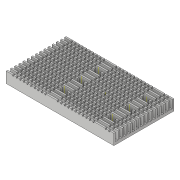
# Autodesk Inventor part: 6089-107-RevA_HEATSINK_VU7P
Saved by Autodesk Inventor 2017.3 (Build 213256000, 256)
## iProperties
Created: 2019-01-23
Part Number: 6089-107-RevA_HEATSINK_VU7P
Material: Generic
Document SubType Name: Modeling
Designer: crs5
Density: 1 g/cm^3
Appearance: Default
Author: crs5
Autodesk Inventor part; units mm, degrees
ref_plane "YZ Plane" through (0, 0, 0) normal (1, 0, 0) x (0, 1, 0)
ref_plane "XZ Plane" through (0, 0, 0) normal (0, 1, 0) x (-1, 0, 0)
ref_plane "XY Plane" through (0, 0, 0) normal (0, 0, 1) x (1, 0, 0)
sketch "Sketch1" plane through (0, 0, 0) normal (0, 1, 0) x (-1, 0, 0)
  line L0 (0, 0) -> (150, 0)
  line L1 (150, 0) -> (150, -83.5)
  line L2 (150, -83.5) -> (0, -83.5)
  line L3 (0, -83.5) -> (0, 0)
  dimension "d0" = 83.5
  dimension "d1" = 150
  constraints: 8 end point, 2 parallel, 1 horizontal, 1 perpendicular
  measures "d0" distance of L2.end L0.start
  measures "d1" distance of L0.start L0.end
extrude "Extrusion1" add sketch "Sketch1" along normal blind 15
hole "Hole1" at (-20, 15, -18.5214) direction (0, -1, 0) diameter 6 end through all counterbore diameter 8.9 counterbore depth 13.5
pattern_linear "Rectangular Pattern1" count 3 spacing 23.2286 along (0, 0, -1) count 2 spacing 67 along (-1, 0, 0) of "Hole1"
hole "Hole2" at (-53.5, 15, -41.75) direction (0, -1, 0) diameter 1.8 end through all
sketch "Sketch2" plane through (0, 0, 0) normal (1, 0, 0) x (0, 0, -1)
  line L0 (0, 15) -> (83.5, 15) projected
  line L1 (2.2, 15) -> (5.8071, 15)
  line L2 (5.8071, 15) -> (5.8071, 4)
  line L3 (5.8071, 4) -> (2.2, 4)
  line L4 (2.2, 4) -> (2.2, 15)
  line L5 (83.5, 0) -> (0, 0) projected
  line L6 (0, 0) -> (0, 15) projected
  dimension "d28" = 4
  dimension "d29" = 2.2
  dimension "d30" = 3.6071
  constraints: 8 end point, 2 parallel, 1 horizontal, 1 perpendicular, 1 point on line
  measures "d28" distance between parallel lines of L5 L3
  measures "d29" distance between parallel lines of L6 L4
  measures "d30" distance of L2.end L3.end
extrude "Extrusion2" cut sketch "Sketch2" against normal up to next
pattern_linear "Rectangular Pattern2" count 14 spacing 5.8071 along (0, 0, -1) of "Extrusion2"
sketch "Sketch3" plane through (-150, 0, 0) normal (0, 0, 1) x (1, 0, 0)
  line L0 (150, 15) -> (0, 15) projected
  line L1 (120.8, 15) -> (122.3, 15)
  line L2 (122.3, 15) -> (122.3, 13.5)
  line L3 (122.3, 13.5) -> (120.8, 13.5)
  line L4 (120.8, 13.5) -> (120.8, 15)
  line L5 (150, 0) -> (150, 15) projected
  dimension "d36" = 1.5
  dimension "d37" = 1.5
  dimension "d38" = 27.7
  constraints: 8 end point, 2 parallel, 1 horizontal, 1 perpendicular, 1 point on line
  measures "d36" distance of L1.end L2.end
  measures "d37" distance of L2.end L3.end
  measures "d38" distance between parallel lines of L2 L5
extrude "Extrusion3" cut sketch "Sketch3" against normal blind 83.5
pattern_linear "Rectangular Pattern3" count 11 spacing 5 along (-1, 0, 0) of "Extrusion3"
sketch "Sketch4" plane through (-150, 0, 0) normal (0, 0, 1) x (1, 0, 0)
  line L0 (150, 15) -> (122.3, 15) projected
  line L1 (137.7, 15) -> (139.2, 15)
  line L2 (139.2, 15) -> (139.2, 13.5)
  line L3 (139.2, 13.5) -> (137.7, 13.5)
  line L4 (137.7, 13.5) -> (137.7, 15)
  line L5 (150, 0) -> (150, 15) projected
  dimension "d44" = 1.5
  dimension "d45" = 1.5
  dimension "d46" = 12.3
  constraints: 8 end point, 2 parallel, 1 horizontal, 1 perpendicular, 1 point on line
  measures "d44" distance of L1.end L2.end
  measures "d45" distance of L2.end L3.end
  measures "d46" distance between parallel lines of L5 L4
extrude "Extrusion4" cut sketch "Sketch4" against normal blind 83.5
pattern_linear "Rectangular Pattern4" count 2 spacing 5 along (1, 0, 0) of "Extrusion4"
sketch "Sketch6" plane through (-150, 0, 0) normal (0, 0, 1) x (1, 0, 0)
  line L0 (0, 15) -> (70.8, 15) projected
  line L1 (53.8, 15) -> (55.3, 15)
  line L2 (55.3, 15) -> (55.3, 13.5)
  line L3 (55.3, 13.5) -> (53.8, 13.5)
  line L4 (53.8, 13.5) -> (53.8, 15)
  line L5 (150, 0) -> (150, 15) projected
  dimension "d52" = 1.5
  dimension "d53" = 1.5
  dimension "d54" = 94.7
  constraints: 8 end point, 2 parallel, 1 horizontal, 1 perpendicular, 1 point on line
  measures "d52" distance of L1.end L2.end
  measures "d53" distance of L2.end L3.end
  measures "d54" distance between parallel lines of L5 L2
extrude "Extrusion5" cut sketch "Sketch6" against normal blind 83.5
pattern_linear "Rectangular Pattern5" count 10 spacing 5 along (-1, 0, 0) of "Extrusion5"
equation "\"d0\" = hs_width"
equation "\"d1\" = hs_length_VU7P"
equation "\"d2\" = hs_overall_height"
equation "\"d6\" = hole_dia"
equation "\"d4\" = hole_ll_x"
equation "\"d5\" = hole_ll_y"
equation "\"d8\" = spring_hole_ID"
equation "\"d9\" = spring_hole_total_depth"
equation "\"d15\" = hole_lc_x - hole_ll_x"
equation "\"d18\" = hole_ul_y - hole_ll_y"
equation "\"d19\" = hole_fpga_center_x"
equation "\"d20\" = hole_fpga_center_y"
equation "\"d23\" = spring_hole_ID"
equation "\"d24\" = spring_hole_total_depth"
equation "\"d28\" = hs_base_thickness"
equation "\"d29\" = hs_fin_thickness"
equation "\"d30\" = hs_fin_gap"
equation "\"d31\" = hs_overall_height"
equation "\"d35\" = hs_pitch"
equation "\"d39\" = hs_width"
equation "\"d47\" = hs_width"
equation "\"d55\" = hs_width"
equation "\"hs_length_VU7P\" = 150"
equation "\"hs_length_KU15P\" = 125"
equation "\"hs_width\" = 83.5"
equation "\"hs_base_thickness\" = 4"
equation "\"hs_overall_height\" = 15"
equation "\"hs_fin_thickness\" = 2.2"
equation "\"hole_y_spacing\" = 67"
equation "\"hole_dia\" = 6"
equation "\"spring_OD\" = 7.9"
equation "\"spring_free_length\" = 9.7"
equation "\"spring_compressed_length\" = 4.8"
equation "\"spring_OD_clearance\" = 1"
equation "\"spring_insertion_depth\" = 2.5"
equation "\"hs_fin_gap\" = 3.60714"
equation "\"hs_pitch\" = 5.80714"
equation "\"hs_center_offset\" = 0"
equation "\"hole_x_spacing\" = 23.22857"
equation "\"hole_ll_x\" = 18.52143"
equation "\"hole_ll_y\" = 20"
equation "\"hole_lc_x\" = 41.75"
equation "\"hole_lr_x\" = 64.97857"
equation "\"hole_ul_x\" = 18.52143"
equation "\"hole_ul_y\" = 87"
equation "\"hole_uc_x\" = 41.75"
equation "\"hole_uc_y\" = 87"
equation "\"hole_ur_x\" = 64.97857"
equation "\"hole_ur_y\" = 87"
equation "\"hole_fpga_center_x\" = 41.75"
equation "\"hole_fpga_center_y\" = 53.5"
equation "\"spring_hole_ID\" = 8.9"
equation "\"spring_hole_total_depth\" = 13.5"
body "Solid1"
